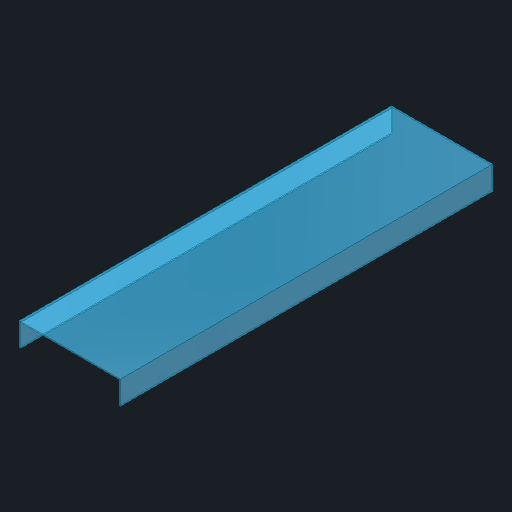
# Autodesk Inventor part: Proteção
Saved by Autodesk Inventor 2026.2 (Build 302298010, 298A)
## iProperties
Created: 2026-03-03
Part Number: Proteção
Material: Polycarbonate, Clear
Document SubType Name: Modeling
Designer: Rubens
Density: 1.2 g/cm^3
Appearance: Polycarbonate - Clear(1)
Author: Rubens
Autodesk Inventor part; units mm, degrees
ref_plane "YZ Plane" through (0, 0, 0) normal (1, 0, 0) x (0, 1, 0)
ref_plane "XZ Plane" through (0, 0, 0) normal (0, 1, 0) x (-1, 0, 0)
ref_plane "XY Plane" through (0, 0, 0) normal (0, 0, 1) x (1, 0, 0)
sketch "Sketch1" plane through (0, 0, 0) normal (0, 0, 1) x (1, 0, 0)
  line L0 (0, 0) -> (0, 100)
  line L1 (0, 100) -> (440, 100)
  line L2 (440, 100) -> (440, 0)
  line L3 (445, 0) -> (445, 105)
  line L4 (445, 105) -> (-5, 105)
  line L5 (-5, 105) -> (-5, 0)
  line L6 (-5, 0) -> (0, 0)
  line L7 (445, 0) -> (440, 0)
  dimension "d1" = 440
  dimension "d4" = 100
  dimension "d5" = 440
  dimension "d6" = 5
  constraints: 16 end point, 2 perpendicular, 1 collinear, 1 horizontal, 1 vertical, 2 other
  measures "d1" distance of L0.start L2.end
  measures "d4" distance of L0.start L0.end
  measures "d5" distance of L0.end L1.end
  measures "d6" distance between parallel lines of L1 L4
extrude "Extrusion1" add sketch "Sketch1" against normal blind 1655
body "Solid1"
